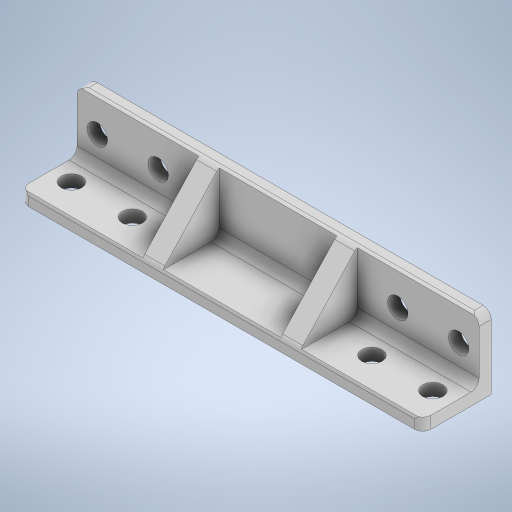
# Autodesk Inventor part: BP_L-Long
Saved by Autodesk Inventor 2024.3 (Build 283343000, 343)
## iProperties
Created: 2025-10-31
Part Number: BP_L-Long
Material: 一般
Document SubType Name: Modeling
Designer: 佐藤智貴
Density: 1 g/cm^3
Appearance: 既定
Author: 佐藤智貴
Autodesk Inventor part; units mm, degrees
ref_plane "YZ Plane" through (0, 0, 0) normal (1, 0, 0) x (0, 1, 0)
ref_plane "XZ Plane" through (0, 0, 0) normal (0, 1, 0) x (-1, 0, 0)
ref_plane "XY Plane" through (0, 0, 0) normal (0, 0, 1) x (1, 0, 0)
sketch "スケッチ1" plane through (0, 0, 0) normal (0, 0, 1) x (1, 0, 0)
  line L0 (0, 0) -> (99, 0)
  line L1 (99, 0) -> (99, 3)
  line L2 (99, 3) -> (0, 3)
  line L3 (0, 3) -> (0, 0)
  dimension "d0" = 3
  dimension "d1" = 99
  constraints: 8 end point, 2 parallel, 1 horizontal, 1 perpendicular
  measures "d0" distance of L0.end L1.end
  measures "d1" distance between parallel lines of L3 L1
extrude "押し出し1" add sketch "スケッチ1" along normal blind 16.9
sketch "スケッチ2" plane through (0, 3, 0) normal (0, 1, 0) x (1, 0, 0)
  line L0 (0, 0) -> (0, -16.9) projected
  line L1 (99, 0) -> (99, -16.9) projected
  line L2 (0, 0) -> (99, 0)
  line L3 (99, 0) -> (99, -3)
  line L4 (99, -3) -> (0, -3)
  line L5 (0, -3) -> (0, 0)
  point P0 (0, -3)
  dimension "d4" = 3
  constraints: 8 end point, 2 parallel, 1 horizontal, 1 perpendicular, 1 point on line
  measures "d4" distance between parallel lines of L2 L4
extrude "押し出し2" add sketch "スケッチ2" along normal blind 15
sketch "スケッチ3" plane through (0, 3, 16.9) normal (0, 1, 0) x (1, 0, 0)
  line L0 (0, 13.9) -> (99, 13.9) projected
  line L1 (99, 13.9) -> (99, 0) projected
  line L2 (99, 0) -> (0, 0) projected
  line L3 (49.5, 0) -> (49.5, 13.9)
  point P0 (0, 16.9)
  point P1 (79, 7.5)
  point P2 (94, 7.5)
  point P3 (20, 7.5)
  point P4 (5, 7.5)
  dimension "d7" = 15
  dimension "d8" = 6.4
  dimension "d9" = 6.4
  dimension "d10" = 5
  constraints: 2 end point, 2 midpoint, 2 symmetric about line
  measures "d7" distance of point (94, 7.5) point (79, 7.5)
  measures "d8" distance from line of L0 point (79, 7.5)
  measures "d9" distance from line of L0 point (94, 7.5)
  measures "d10" distance from line of L1 point (94, 7.5)
hole "穴1" at (79, 3, 9.4) at (94, 3, 9.4) at (5, 3, 9.4) at (20, 3, 9.4) direction (0, -1, 0) diameter 5 end through all
sketch "スケッチ4" plane through (0, 3, 3) normal (0, 0, 1) x (1, 0, 0)
  line L0 (99, 0) -> (0, 0) projected
  line L1 (0, 0) -> (0, 15) projected
  line L2 (49.5, 0) -> (49.5, 15)
  line L3 (0, 15) -> (99, 15) projected
  point P0 (0, -3)
  point P1 (5, 7)
  point P2 (20, 7)
  point P3 (94, 7)
  point P4 (79, 7)
  dimension "d18" = 7
  dimension "d19" = 7
  dimension "d20" = 15
  dimension "d21" = 5
  constraints: 2 end point, 2 midpoint, 2 symmetric about line
  measures "d18" distance from line of L0 point (20, 7)
  measures "d19" distance from line of L0 point (5, 7)
  measures "d20" distance of point (20, 7) point (5, 7)
  measures "d21" distance from line of L1 point (5, 7)
hole "穴2" at (5, 10, 3) at (20, 10, 3) at (79, 10, 3) at (94, 10, 3) direction (0, 0, -1) diameter 5 end through all
sketch "スケッチ7" plane through (0, 3, 16.9) normal (0, 1, 0) x (1, 0, 0)
  line L0 (99, 13.9) -> (0, 13.9) projected
  line L1 (99, 0) -> (0, 0) projected
  line L2 (64, 13.9) -> (69, 13.9)
  line L3 (69, 13.9) -> (69, 0)
  line L4 (69, 0) -> (64, 0)
  line L5 (64, 0) -> (64, 13.9)
  line L6 (99, 13.9) -> (99, 0) projected
  line L7 (30, 13.9) -> (35, 13.9)
  line L8 (35, 13.9) -> (35, 0)
  line L9 (35, 0) -> (30, 0)
  line L10 (30, 0) -> (30, 13.9)
  line L11 (0, 13.9) -> (0, 0) projected
  point P0 (0, 16.9)
  point P1 (64, 0)
  point P2 (69, 13.9)
  point P3 (30, 0)
  dimension "d36" = 5
  dimension "d37" = 30
  dimension "d43" = 5
  dimension "d44" = 30
  constraints: 16 end point, 4 parallel, 4 point on line, 2 horizontal, 2 perpendicular
  measures "d36" distance between parallel lines of L3 L5
  measures "d37" distance between parallel lines of L6 L3
  measures "d43" distance between parallel lines of L10 L8
  measures "d44" distance between parallel lines of L11 L10
extrude "押し出し5" add sketch "スケッチ7" along normal blind 15 contours L3 L1 L5 L0 | L8 L1 L10 L0
sketch "スケッチ8" plane through (64, 3, 3) normal (-1, 0, 0) x (0, 0, 1)
  line L0 (13.9, 0) -> (0, 0) projected
  line L1 (13.9, 0) -> (13.9, 15) projected
  line L2 (0, 15) -> (13.9, 15) projected
  line L3 (0, 0) -> (0, 15) projected
  line L4 (13.9, 0) -> (0, 15)
  point P0 (-3, -3)
  constraints: 2 end point
extrude "押し出し6" cut sketch "スケッチ8" along normal blind 200 and the other way blind 7.5 contours L4 L2 L1
fillet "フィレット1" radius 2 9 edges at (0, 18, 1.5) (99, 18, 1.5) (99, 1.5, 16.9) (0, 1.5, 16.9) (84, 3, 3) (15, 3, 3) (49.5, 3, 3) (66.5, 18, 3) (66.5, 3, 16.9)
equation "\"d9\" = d8"
equation "\"d19\" = d18"
equation "\"d43\" = d36"
equation "\"d44\" = d37"
